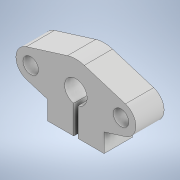
# Autodesk Inventor part: SHF08
Saved by Autodesk Inventor 2020 (Build 240168000, 168)
## iProperties
Created: 2022-03-20
Part Number: SHF08
Material: Generic
Document SubType Name: Modeling
Designer: Admin
Density: 1 g/cm^3
Appearance: Default
Author: Admin
Autodesk Inventor part; units mm, degrees
ref_plane "YZ Plane" through (0, 0, 0) normal (1, 0, 0) x (0, 1, 0)
ref_plane "XZ Plane" through (0, 0, 0) normal (0, 1, 0) x (-1, 0, 0)
ref_plane "XY Plane" through (0, 0, 0) normal (0, 0, 1) x (1, 0, 0)
sketch "Sketch1" plane through (0, 0, 0) normal (0, 0, 1) x (1, 0, 0)
  circle A0 centre (-16, 0) radius 2.75
  circle A1 centre (16, 0) radius 2.75
  circle A2 centre (0, 0) radius 4
  circle A3 centre (-16, 0) radius 5.25
  circle A4 centre (16, 0) radius 5.25
  circle A5 centre (0, 0) radius 10
  line L0 (-2.9687, 9.5492) -> (-17.5586, 5.0133)
  line L1 (2.9687, 9.5492) -> (17.5586, 5.0133)
  line L2 (-17.5586, -5.0133) -> (-2.9688, -9.5492)
  line L3 (2.9687, -9.5492) -> (17.5586, -5.0133)
  line L4 (-10, 3.0548) -> (10, 3.0548)
  line L5 (10, 3.0548) -> (10, -14)
  line L6 (10, -14) -> (-10, -14)
  line L7 (-10, -14) -> (-10, 3.0548)
  line L8 (-0.75, 0) -> (0.75, 0)
  line L9 (0.75, 0) -> (0.75, -14)
  line L10 (0.75, -14) -> (-0.75, -14)
  line L11 (-0.75, -14) -> (-0.75, 0)
  point P0 (-9.522, 3.0548)
  point P1 (-10, 0)
  point P2 (-10, -7.3632)
  point P3 (-0.75, -3.9291)
  point P4 (0.75, -3.9291)
  point P5 (10, -7.3632)
  point P6 (9.522, 3.0548)
  point P7 (10, 0)
  dimension "d0" = 5.5
  dimension "d1" = 5.5
  dimension "d2" = 32
  dimension "d3" = 16
  dimension "d4" = 8
  dimension "d5" = 10.5
  dimension "d6" = 10.5
  dimension "d7" = 20
  dimension "d8" = 0
  dimension "d9" = 0
  dimension "d10" = 14
  dimension "d11" = 20
  dimension "d12" = 10
  dimension "d13" = 1.5
  dimension "d14" = 0.75
  constraints: 24 end point, 8 point on circle, 8 tangent, 6 centre point, 4 coincident, 4 parallel, 2 horizontal, 2 perpendicular, 1 point on line
  measures "d0" diameter of A0
  measures "d1" diameter of A1
  measures "d2" distance of A1.centre A0.centre
  measures "d3" distance of A0.centre point (0, 0)
  measures "d4" diameter of A2
  measures "d5" diameter of A3
  measures "d6" diameter of A4
  measures "d7" diameter of A5
  measures "d8" vertical distance of A0.centre point (0, 0)
  measures "d9" vertical distance of point (0, 0) A1.centre
  measures "d10" distance from line of L6 point (0, 0)
  measures "d11" distance between parallel lines of L5 L7
  measures "d12" distance from line of L7 A2.centre
  measures "d13" distance of L9.end L10.end
  measures "d14" distance from line of L11 point (0, 0)
extrude "Extrusion1" add sketch "Sketch1" along normal blind 10 contours A2 L4 A5 L9 | A2 L4 A5 | A2 L11 A5 L4 | L4 L5 A5 | A5 L1 A4 L3 L5 L4 | A5 L3 L5 L6 L9 | L4 L7 L2 A3 L0 A5 | A5 L7 L4 | L5 L3 A5 | L11 L6 L7 L2 A5 | A5 L2 L7 | A4 | A3
body "Solid1"
